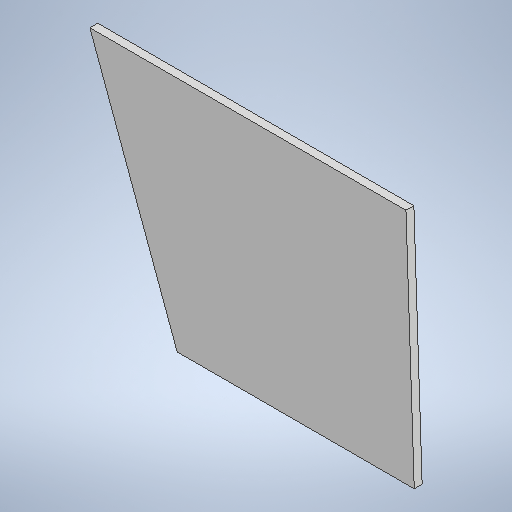
# Autodesk Inventor part: полка под швеллер
Saved by Autodesk Inventor 2025 (Build 290162010, 162A)
## iProperties
Created: 2024-06-15
Part Number: полка под швеллер
Material: Generic
Document SubType Name: Sheet Metal
Designer: admin
Density: 1 g/cm^3
Sheet Metal Rule: Default
Appearance: Default
Author: admin
Autodesk Inventor part; units mm, degrees
ref_plane "YZ Plane" through (0, 0, 0) normal (1, 0, 0) x (0, 1, 0)
ref_plane "XZ Plane" through (0, 0, 0) normal (0, 1, 0) x (-1, 0, 0)
ref_plane "XY Plane" through (0, 0, 0) normal (0, 0, 1) x (1, 0, 0)
sketch "Sketch5" plane through (0, 0, 0) normal (0, 1, 0) x (-1, 0, 0)
  line L0 (200, 0) -> (-200, 0)
  line L1 (-210.4762, -300) -> (89.5238, -300)
  line L2 (89.5238, -300) -> (200, 0)
  line L3 (-200, 0) -> (-210.4762, -300)
  line L4 (-200, 0) -> (-200, -300) construction
  point P0 (0, 0)
  point P1 (0, 0)
  dimension "d26" = 400
  dimension "d27" = 2
  dimension "d28" = 300
  dimension "d29" = 300
  measures "d26" distance of L0.start L0.end
  measures "d27" angle of L4 L3
  measures "d28" distance of L1.start L1.end
  measures "d29" distance between parallel lines of L1 L0
extrude "Plate3" add sketch "Sketch5" along normal blind 10
equation "\"d30\" = Thickness"
equation "\"BendReliefDepth\" = 0.5 * Thickness"
equation "\"Thickness\" = 10"
body "Solid2"
